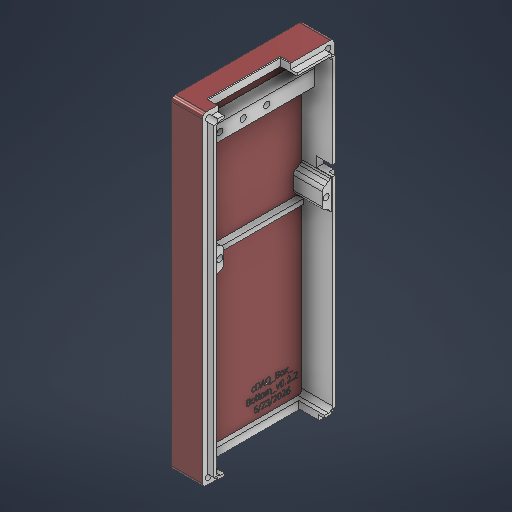
# Autodesk Inventor part: cDAQ_Box_Bottom_v0.2.2ipt
Saved by Autodesk Inventor 2027 (Build 310192000, 192)
## iProperties
Created: 2026-05-08
Part Number: cDAQ_Box_Bottom_v0.2.2ipt
Material: Generic
Document SubType Name: Modeling
Designer: giese
Density: 1 g/cm^3
Appearance: Default
Author: giese
Autodesk Inventor part; units mm, degrees
(part 1 of 2)
ref_plane "YZ Plane" through (0, 0, 0) normal (1, 0, 0) x (0, 1, 0)
ref_plane "XZ Plane" through (0, 0, 0) normal (0, 1, 0) x (-1, 0, 0)
ref_plane "XY Plane" through (0, 0, 0) normal (0, 0, 1) x (1, 0, 0)
sketch "Sketch1" plane through (0, 0, 0) normal (1, 0, 0) x (0, 1, 0)
  line L0 (37.5698, 55.7067) -> (-217.4462, 55.7067)
  line L1 (-217.4462, 55.7067) -> (-217.4462, -48.4333)
  line L2 (-217.4462, -48.4333) -> (37.5698, -48.4333)
  line L3 (37.5698, -48.4333) -> (37.5698, 55.7067)
  point P0 (0, 0)
  dimension "d0" = 104.14
  dimension "d1" = 255.016
  constraints: 8 end point, 2 parallel, 1 horizontal, 1 perpendicular
  measures "d0" distance of L2.end L0.start
  measures "d1" distance of L1.end L2.end
extrude "Extrusion1" add sketch "Sketch1" along normal blind 24.13
sketch "Sketch2" plane through (24.13, 0, 0) normal (1, 0, 0) x (0, 0, -1)
  line L0 (42.0833, 31.2198) -> (-49.3567, 31.2198)
  line L1 (-49.3567, 31.2198) -> (-49.3567, -211.0962)
  line L2 (-49.3567, -211.0962) -> (42.0833, -211.0962)
  line L3 (42.0833, -211.0962) -> (42.0833, 31.2198)
  line L4 (48.4333, 37.5698) -> (-55.7067, 37.5698) projected
  line L5 (-55.7067, 37.5698) -> (-55.7067, -217.4462) projected
  line L6 (-55.7067, -217.4462) -> (48.4333, -217.4462) projected
  line L7 (48.4333, -217.4462) -> (48.4333, 37.5698) projected
  point P0 (0, 0)
  dimension "d4" = 242.316
  dimension "d5" = 91.44
  dimension "d8" = 6.35
  dimension "d21" = 6.35
  dimension "d690" = 6.35
  dimension "d842" = 6.35
  constraints: 8 end point, 2 parallel, 1 horizontal, 1 perpendicular
  measures "d4" distance of L2.end L0.start
  measures "d5" distance of L0.start L0.end
  measures "d8" distance between parallel lines of L0 L4
  measures "d21" distance between parallel lines of L5 L1
  measures "d690" distance between parallel lines of L6 L2
  measures "d842" distance between parallel lines of L7 L3
extrude "Extrusion2" cut sketch "Sketch2" against normal blind 19.05 contours L3 L2 L1 L0
sketch "Sketch3" plane through (0, 0, 0) normal (-1, 0, 0) x (0, 0, 1)
  circle A0 centre (-4.1509, 9.6298) radius 2.4005
  circle A1 centre (14.3479, 9.6298) radius 2.4005
  circle A2 centre (32.8467, 9.6298) radius 2.4005
  line L0 (-48.4333, -217.4462) -> (-48.4333, 37.5698) projected
  line L1 (-48.4333, 37.5698) -> (55.7067, 37.5698) projected
  line L2 (55.7067, 37.5698) -> (55.7067, -217.4462) projected
  line L3 (49.3567, 31.2198) -> (-42.0833, 31.2198) projected
  point P0 (0, 0)
  point P1 (-0.896, -23.7433)
  point P2 (-45.1848, 27.0137)
  dimension "d9" = 18.4988
  dimension "d10" = 4.801
  dimension "d11" = 4.801
  dimension "d12" = 18.4988
  dimension "d13" = 36.9976
  dimension "d18" = 22.86
  dimension "d22" = 4.801
  dimension "d58" = 27.94
  constraints: 3 centre point
  measures "d9" distance of A0.centre A1.centre
  measures "d10" diameter of A1
  measures "d11" diameter of A2
  measures "d12" distance of A1.centre A2.centre
  measures "d13" distance of A0.centre A2.centre
  measures "d18" distance from line of L2 A2.centre
  measures "d22" diameter of A0
  measures "d58" distance from line of L1 A2.centre
extrude "Extrusion3" cut sketch "Sketch3" against normal blind 5.08
sketch "Sketch5" plane through (0, -217.4462, -48.4333) normal (0, 0, -1) x (-1, 0, 0)
  line L0 (-27.2034, 165.862) -> (-16.51, 165.862)
  line L1 (-16.51, 165.862) -> (-16.51, 173.862)
  line L2 (-16.51, 173.862) -> (-27.2034, 173.862)
  line L3 (-27.2034, 173.862) -> (-27.2034, 165.862)
  line L4 (0, 255.016) -> (-24.13, 255.016) projected
  line L5 (0, 0) -> (0, 255.016) projected
  line L6 (-24.13, 0) -> (-24.13, 255.016) projected
  line L7 (0, 0) -> (-24.13, 0) projected
  point P0 (0, 217.4462)
  point P1 (-21.8567, 173.862)
  point P2 (-21.8567, 165.862)
  dimension "d28" = 10.6934
  dimension "d30" = 8
  dimension "d31" = 16.51
  dimension "d215" = 3.0734
  dimension "d1133" = 165.862
  constraints: 8 end point, 2 midpoint, 2 parallel, 1 horizontal, 1 perpendicular
  measures "d28" distance between parallel lines of L1 L3
  measures "d30" distance of point (-21.857, 173.862) point (-21.857, 165.862)
  measures "d31" distance between parallel lines of L5 L1
  measures "d215" distance between parallel lines of L6 L3
  measures "d1133" distance between parallel lines of L7 L0
extrude "Extrusion4" cut sketch "Sketch5" against normal blind 24.13 contours L3 L2 L6 L0 | L6 L2 L1 L0
sketch "Sketch6" plane through (0, -217.4462, -48.4333) normal (0, -1, 0) x (1, 0, 0)
  line L0 (24.08, 55.136) -> (16.08, 55.136)
  line L1 (16.08, 45.136) -> (24.08, 45.136)
  line L2 (0, 104.14) -> (0, 0) projected
  line L3 (29.63, 53.1359) -> (29.63, 47.136)
  line L4 (24.08, 55.136) -> (29.63, 53.1359)
  line L5 (29.63, 47.136) -> (24.08, 45.136)
  line L6 (0, 0) -> (24.13, 0) projected
  line L7 (24.13, 97.79) -> (24.13, 6.35) projected
  line L8 (24.13, 41.9134) -> (24.13, 37.4697)
  line L9 (16.08, 55.136) -> (8.636, 55.136)
  line L10 (8.636, 55.136) -> (8.636, 45.136)
  line L11 (8.636, 45.136) -> (21.16, 45.136)
  point P0 (0, 48.4333)
  point P1 (20.08, 55.136)
  point P2 (20.08, 45.136)
  point P3 (16.08, 50.136)
  dimension "d39" = 6
  dimension "d48" = 55.136
  dimension "d221" = 0
  dimension "d223" = 2
  dimension "d224" = 2
  dimension "d225" = 5.5
  dimension "d227" = 5.55
  dimension "d672" = 8.636
  constraints: 18 end point, 2 horizontal, 2 midpoint, 2 parallel, 2 point on line, 1 perpendicular, 1 vertical
  measures "d39" distance of L3.start L3.end
  measures "d48" distance between parallel lines of L6 L0
  measures "d221" horizontal distance of L0.start L1.end
  measures "d223" vertical distance of L3.end L1.end
  measures "d224" vertical distance of L0.start L3.start
  measures "d225" distance between parallel lines of L3 L7
  measures "d227" distance from line of L1.end L3
  measures "d672" distance between parallel lines of L2 L10
extrude "Extrusion5" [suppressed]
sketch "Sketch7" plane through (0, 37.5698, 55.7067) normal (0, 1, 0) x (1, 0, 0)
  line L0 (31.0134, 69.85) -> (16.002, 69.85)
  line L1 (16.002, 69.85) -> (16.002, 12.7)
  line L2 (16.002, 12.7) -> (31.0134, 12.7)
  line L3 (31.0134, 12.7) -> (31.0134, 69.85)
  line L4 (0, 0) -> (24.13, 0) projected
  line L5 (0, 104.14) -> (0, 0) projected
  line L6 (24.13, 104.14) -> (24.13, 0) projected
  point P0 (0, 55.7067)
  point P1 (24.13, 69.85)
  point P2 (24.13, 12.7)
  dimension "d52" = 12.7
  dimension "d55" = 16.002
  dimension "d56" = 15.0114
  dimension "d57" = 6.8834
  dimension "d1195" = 69.85
  constraints: 8 end point, 2 parallel, 1 horizontal, 1 perpendicular
  measures "d52" distance between parallel lines of L4 L2
  measures "d55" distance between parallel lines of L5 L1
  measures "d56" distance between parallel lines of L3 L1
  measures "d57" distance between parallel lines of L6 L3
  measures "d1195" distance between parallel lines of L4 L0
extrude "Extrusion6" cut sketch "Sketch7" against normal blind 7.62
fillet "Fillet1" radius 3.175 4 edges at (12.065, 37.5698, -48.4333) (12.065, 37.5698, 55.7067) (12.065, -217.4462, -48.4333) (12.065, -217.4462, 55.7067)
sketch "Sketch8" plane through (0, 0, 0) normal (-1, 0, 0) x (0, 0, 1)
  line L0 (-5.9225, 6.0992) -> (-2.3919, 6.0992)
  line L1 (-5.9225, 13.1604) -> (-2.3919, 13.1604)
  line L2 (-5.9225, 6.0992) -> (-7.9609, 9.6298)
  line L3 (-5.9225, 13.1604) -> (-7.9609, 9.6298)
  line L4 (-2.3919, 6.0992) -> (-0.3536, 9.6298)
  line L5 (-2.3919, 13.1604) -> (-0.3536, 9.6298)
  circle A0 centre (-4.1509, 9.6298) radius 2.4005 projected
  line L6 (12.5763, 6.0992) -> (16.1069, 6.0992)
  line L7 (12.5763, 13.1604) -> (16.1069, 13.1604)
  line L8 (12.5763, 6.0992) -> (10.5379, 9.6298)
  line L9 (12.5763, 13.1604) -> (10.5379, 9.6298)
  line L10 (16.1069, 6.0992) -> (18.1453, 9.6298)
  line L11 (16.1069, 13.1604) -> (18.1453, 9.6298)
  circle A1 centre (14.3479, 9.6298) radius 2.4005 projected
  line L12 (31.0751, 6.0992) -> (29.0367, 9.6298)
  line L13 (31.0751, 13.1604) -> (29.0367, 9.6298)
  line L14 (31.0751, 6.0992) -> (34.6057, 6.0992)
  line L15 (31.0751, 13.1604) -> (34.6057, 13.1604)
  line L16 (34.6057, 6.0992) -> (36.6441, 9.6298)
  line L17 (34.6057, 13.1604) -> (36.6441, 9.6298)
  circle A2 centre (32.8467, 9.6298) radius 2.4005 projected
  point P0 (-4.1572, 6.0992)
  point P1 (14.3416, 6.0992)
  point P2 (32.8404, 6.0992)
  point P3 (-7.9609, 9.6298)
  point P4 (-0.3536, 9.6298)
  point P5 (18.1453, 9.6298)
  point P6 (10.5379, 9.6298)
  point P7 (36.6441, 9.6298)
  point P8 (29.0367, 9.6298)
  dimension "d60" = 7.0612
  dimension "d61" = 120
  dimension "d62" = 120
  dimension "d63" = 120
  dimension "d64" = 120
  dimension "d65" = 3.5306
  dimension "d66" = 3.5306
  dimension "d67" = 3.5306
  dimension "d68" = 3.5306
  dimension "d69" = 3.5306
  dimension "d70" = 3.5306
  dimension "d71" = 0
  dimension "d72" = 7.6074
  dimension "d73" = 3.81
  dimension "d74" = 0
  dimension "d75" = 7.0612
  dimension "d76" = 120
  dimension "d77" = 120
  dimension "d78" = 120
  dimension "d79" = 120
  dimension "d80" = 3.5306
  dimension "d81" = 3.5306
  dimension "d82" = 3.5306
  dimension "d83" = 3.5306
  dimension "d84" = 3.5306
  dimension "d85" = 3.5306
  dimension "d86" = 0
  dimension "d87" = 7.6074
  dimension "d91" = 0
  dimension "d92" = 3.81
  dimension "d93" = 7.0612
  dimension "d94" = 120
  dimension "d95" = 120
  dimension "d96" = 120
  dimension "d97" = 120
  dimension "d98" = 3.5306
  dimension "d99" = 3.5306
  dimension "d100" = 3.5306
  dimension "d101" = 3.5306
  dimension "d102" = 3.5306
  dimension "d103" = 3.5306
  dimension "d104" = 0
  dimension "d105" = 7.6074
  dimension "d108" = 0
  dimension "d109" = 3.81
  constraints: 36 end point, 6 horizontal, 3 midpoint
  measures "d60" distance from line of point (-4.157, 6.099) L1
  measures "d61" angle of L0 L2
  measures "d62" angle of L1 L3
  measures "d63" angle of L4 L0
  measures "d64" angle of L5 L1
  measures "d65" distance of L0.start L0.end
  measures "d66" distance of L1.start L1.end
  measures "d67" vertical distance of L1.start L3.end
  measures "d68" vertical distance of L0.start L2.end
  measures "d69" vertical distance of L1.end L5.end
  measures "d70" vertical distance of L0.end L4.end
  measures "d71" horizontal distance of L0.start L1.start
  measures "d72" distance of L4.end L2.end
  measures "d73" distance of A0.centre L2.end
  measures "d74" vertical distance of A0.centre L4.end
  measures "d75" distance from line of point (14.342, 6.099) L7
  measures "d76" angle of L6 L8
  measures "d77" angle of L7 L9
  measures "d78" angle of L10 L6
  measures "d79" angle of L11 L7
  measures "d80" distance of L8.start L6.end
  measures "d81" distance of L9.start L7.end
  measures "d82" vertical distance of L9.start L9.end
  measures "d83" vertical distance of L8.start L8.end
  measures "d84" vertical distance of L7.end L11.end
  measures "d85" vertical distance of L6.end L10.end
  measures "d86" horizontal distance of L8.start L9.start
  measures "d87" distance of L10.end L8.end
  measures "d91" vertical distance of A1.centre L8.end
  measures "d92" distance of A1.centre L8.end
  measures "d93" distance from line of point (32.84, 6.099) L15
  measures "d94" angle of L14 L12
  measures "d95" angle of L15 L13
  measures "d96" angle of L16 L14
  measures "d97" angle of L17 L15
  measures "d98" distance of L12.start L16.start
  measures "d99" distance of L15.start L15.end
  measures "d100" vertical distance of L15.start L13.end
  measures "d101" vertical distance of L12.start L12.end
  measures "d102" vertical distance of L15.end L17.end
  measures "d103" vertical distance of L16.start L16.end
  measures "d104" horizontal distance of L12.start L15.start
  measures "d105" distance of L16.end L12.end
  measures "d108" vertical distance of A2.centre L12.end
  measures "d109" distance of A2.centre L12.end
extrude "Extrusion7" cut sketch "Sketch8" against normal blind 4 contours L2 L3 L1 L5 L4 L0 | A0 | L8 L9 L7 L11 L10 L6 | A1 | L12 L13 L15 L17 L16 L14 | A2
sketch "Sketch9" plane through (5.08, 0, 0) normal (1, 0, 0) x (0, 0, -1)
  arc A0 (24.8089, -180.8044) -> (19.3527, -180.8044) centre (22.0808, -178.3302) ccw
  line L0 (45.2583, 37.5698) -> (14.1433, 37.5698) projected
  line L1 (42.0833, 31.2198) -> (42.0833, -43.5842) projected
  arc A1 (20.1758, -185.9502) -> (23.9858, -185.9502) centre (22.0808, -185.9502) ccw
  line L2 (23.9858, -185.9502) -> (23.9858, -182.9374)
  line L3 (20.1758, -185.9502) -> (20.1758, -182.9374)
  arc A2 (24.8089, -180.8044) -> (23.9858, -182.9374) centre (27.1608, -182.9374) ccw
  arc A3 (20.1758, -182.9374) -> (19.3527, -180.8044) centre (17.0008, -182.9374) ccw
  arc A4 (-25.9911, -180.8044) -> (-31.4473, -180.8045) centre (-28.7192, -178.3302) ccw
  arc A5 (-30.6242, -185.9366) -> (-26.8142, -185.9502) centre (-28.7192, -185.9502) ccw
  line L4 (-26.8142, -185.9502) -> (-26.8142, -182.9374)
  line L5 (-30.6242, -185.9366) -> (-30.6242, -182.9374)
  arc A6 (-25.9911, -180.8044) -> (-26.8142, -182.9374) centre (-23.6392, -182.9374) ccw
  arc A7 (-30.6242, -182.9374) -> (-31.4473, -180.8045) centre (-33.7992, -182.9374) ccw
  line L6 (-43.0067, 37.5698) -> (-52.5317, 37.5698) projected
  line L7 (-49.3567, -211.0962) -> (-49.3567, 31.2198) projected
  point P0 (0, 0)
  point P1 (42.0833, -211.0962)
  point P2 (23.9858, -181.4823)
  point P3 (20.1758, -181.4823)
  point P4 (-26.8142, -181.4823)
  point P5 (-30.6242, -181.4823)
  point P6 (-49.3567, 31.2198)
  point P7 (-46.8167, -217.4462)
  dimension "d112" = 215.9
  dimension "d114" = 7.366
  dimension "d116" = 3.81
  dimension "d117" = 223.52
  dimension "d118" = 3.175
  dimension "d119" = 7.366
  dimension "d120" = 3.81
  dimension "d121" = 3.175
  dimension "d122" = 215.9
  dimension "d123" = 223.52
  dimension "d125" = 0
  dimension "d128" = 50.8
  dimension "d129" = 20.0025
  dimension "d130" = 0
  constraints: 20 point on circle, 8 centre point, 8 end point, 8 tangent, 4 point on line, 2 equal radius, 2 parallel, 2 vertical, 1 other
  measures "d112" distance from line of L0 A0.centre
  measures "d114" diameter of A0
  measures "d116" diameter of A1
  measures "d117" distance from line of L0 A1.centre
  measures "d118" radius of A2
  measures "d119" diameter of A4
  measures "d120" diameter of A5
  measures "d121" radius of A6
  measures "d122" distance from line of A4.centre L6
  measures "d123" distance from line of L6 A5.centre
  measures "d125" horizontal distance of A5.centre A4.centre
  measures "d128" distance of A5.centre A1.centre
  measures "d129" distance from line of L1 A0.centre
  measures "d130" horizontal distance of A0.centre A1.centre
extrude "Extrusion8" [suppressed]
sketch "Sketch10" plane through (24.13, 0, 0) normal (1, 0, 0) x (0, 0, -1)
  line L0 (-49.3567, 31.2198) -> (42.0833, 31.2198) projected
  line L1 (-49.3567, 31.2198) -> (42.0833, 31.2198)
  line L2 (42.0833, 33.2264) -> (-46.8167, 33.2264)
  line L3 (-46.8167, 33.2264) -> (-51.3633, 33.2264)
  line L4 (-51.3633, 33.2264) -> (-51.3633, -213.1028)
  line L5 (-51.3633, -213.1028) -> (44.0899, -213.1028)
  line L6 (44.0899, -213.1028) -> (44.0899, 33.2264)
  line L7 (44.0899, 33.2264) -> (41.9392, 33.2264)
  line L8 (42.0833, 31.2198) -> (42.0833, -43.5842) projected
  line L9 (-49.3567, -211.0962) -> (-49.3567, 31.2198) projected
  line L10 (42.0833, -211.0962) -> (-49.3567, -211.0962) projected
  line L11 (45.2583, 37.5698) -> (14.1433, 37.5698) projected
  line L12 (42.0833, 31.2198) -> (42.0833, -211.0962)
  line L13 (42.0833, -211.0962) -> (-49.3567, -211.0962)
  line L14 (-52.5317, -217.4462) -> (45.2583, -217.4462) projected
  line L15 (-49.3567, -211.0962) -> (-49.3567, 31.2198)
  line L16 (-49.3567, 31.2198) -> (42.0833, 31.2198)
  point P0 (-46.8167, -217.4462)
  dimension "d202" = 2.0066
  dimension "d203" = 2.0066
  dimension "d204" = 2.0066
  dimension "d205" = 2.0066
  dimension "d208" = 4.3434
  constraints: 22 end point, 5 perpendicular, 3 point on line, 2 parallel, 1 collinear, 1 horizontal, 1 other
  measures "d202" distance between parallel lines of L0 L2
  measures "d203" distance between parallel lines of L6 L8
  measures "d205" distance between parallel lines of L5 L10
  measures "d208" distance between parallel lines of L11 L2
extrude "Extrusion9" add sketch "Sketch10" along normal blind 5
fillet "Fillet2" radius 3.175 8 edges at (17.105, 31.2198, -42.0833) (17.105, 31.2198, 49.3567) (17.105, -211.0962, 49.3567) (17.105, -211.0962, -42.0833) (26.63, 33.2264, -44.0899) (26.63, 33.2264, 51.3633) (26.63, -213.1028, -44.0899) (26.63, -213.1028, 51.3633)
sketch "Sketch13" plane through (29.13, 0, 0) normal (1, 0, 0) x (0, 0, -1)
  arc A0 (44.0833, 30.0448) -> (40.9083, 33.2198) centre (40.9083, 30.0448) ccw projected
  arc A1 (-45.6417, 33.2198) -> (-48.8167, 30.0448) centre (-45.6417, 30.0448) ccw projected
  arc A2 (40.9083, -212.0802) -> (44.0833, -208.9052) centre (40.9083, -208.9052) ccw projected
  arc A3 (-48.8167, -208.9052) -> (-45.6417, -212.0802) centre (-45.6417, -208.9052) ccw projected
  line L0 (-43.0067, 37.5698) -> (-52.5317, 37.5698) projected
  line L1 (-55.7067, 34.3948) -> (-55.7067, -214.2712) projected
  line L2 (-52.5317, -217.4462) -> (45.2583, -217.4462) projected
  arc A4 (-48.8167, -208.9052) -> (-45.6417, -212.0802) centre (-45.6417, -208.9052) ccw projected
  circle A5 centre (-50.6267, -212.3662) radius 2.4005
  circle A6 centre (43.3533, -212.3662) radius 2.4005
  line L3 (48.4333, -214.2712) -> (48.4333, 34.3948) projected
  circle A7 centre (43.3533, 32.4898) radius 2.4005
  line L4 (45.2583, 37.5698) -> (14.1433, 37.5698) projected
  circle A8 centre (-50.6267, 32.4898) radius 2.4005
  arc A9 (41.4904, -28.6131) -> (38.3154, -25.4381) centre (38.3154, -28.6131) ccw
  circle A10 centre (38.2733, -64.0302) radius 2.4005
  circle A11 centre (-45.5467, -64.0302) radius 2.4005
  point P0 (0, 0)
  point P1 (-47.8868, 32.2898)
  point P2 (-47.8868, -211.1503)
  point P3 (-47.8868, -211.1503)
  point P4 (45.8404, -24.2631)
  point P5 (42.6654, -21.0881)
  dimension "d178" = 5.08
  dimension "d179" = 5.08
  dimension "d180" = 4.801
  dimension "d181" = 5.08
  dimension "d182" = 5.08
  dimension "d183" = 4.801
  dimension "d184" = 4.801
  dimension "d185" = 5.08
  dimension "d186" = 5.08
  dimension "d187" = 4.801
  dimension "d188" = 5.08
  dimension "d189" = 5.08
  dimension "d326" = 4.801
  dimension "d327" = 10.16
  dimension "d328" = 101.6
  dimension "d329" = 4.801
  dimension "d330" = 10.16
  dimension "d331" = 101.6
  constraints: 7 centre point, 5 point on circle
  measures "d178" distance from line of L1 A5.centre
  measures "d179" distance from line of L2 A5.centre
  measures "d180" diameter of A5
  measures "d181" distance from line of L2 A6.centre
  measures "d182" distance from line of L3 A6.centre
  measures "d183" diameter of A6
  measures "d184" diameter of A7
  measures "d185" distance from line of L3 A7.centre
  measures "d186" distance from line of L4 A7.centre
  measures "d187" diameter of A8
  measures "d188" distance from line of L0 A8.centre
  measures "d189" distance from line of L1 A8.centre
  measures "d326" diameter of A10
  measures "d327" distance from line of L3 A10.centre
  measures "d328" distance from line of A10.centre L4
  measures "d329" diameter of A11
  measures "d330" distance from line of L1 A11.centre
  measures "d331" distance from line of L0 A11.centre
extrude "Extrusion11" cut sketch "Sketch13" against normal blind 25.4
sketch "Sketch14" plane through (5.08, 0, 0) normal (1, 0, 0) x (0, 0, -1)
  line L0 (8.8875, -186.6885) -> (28.1042, -186.6885) construction
  line L1 (28.1042, -186.6885) -> (28.1042, -184.7391) construction
  line L2 (28.1042, -184.7391) -> (8.8875, -184.7391) construction
  line L3 (8.8875, -184.7391) -> (8.8875, -186.6885) construction
  spline S0 degree 2 poles (3.9907, -191.4347) (3.635, -191.4347) (3.0459, -191.2161) (2.8347, -190.9938) knots 0 0 0 1 2 2 2
  spline S1 degree 2 poles (2.8347, -190.9938) (2.6236, -190.7752) (2.3901, -190.1008) (2.3901, -189.6488) knots 0 0 0 1 2 2 2
  spline S2 degree 2 poles (2.3901, -189.6488) (2.3901, -189.1968) (2.631, -188.5373) (2.8347, -188.315) knots 0 0 0 1 2 2 2
  spline S3 degree 2 poles (2.8347, -188.315) (3.0385, -188.089) (3.6424, -187.8482) (3.9907, -187.8482) knots 0 0 0 1 2 2 2
  spline S4 degree 2 poles (3.9907, -187.8482) (4.2723, -187.8482) (4.7984, -188.0075) (5.0022, -188.1112) knots 0 0 0 1 2 2 2
  line L4 (5.0022, -188.1112) -> (5.0022, -188.7596)
  line L5 (5.0022, -188.7596) -> (4.9688, -188.7596)
  spline S5 degree 2 poles (4.9688, -188.7596) (4.9058, -188.7078) (4.7132, -188.5744) (4.5761, -188.504) knots 0 0 0 1 2 2 2
  spline S6 degree 2 poles (4.5761, -188.504) (4.4538, -188.4447) (4.1278, -188.3521) (3.9796, -188.3521) knots 0 0 0 1 2 2 2
  spline S7 degree 2 poles (3.9796, -188.3521) (3.5313, -188.3521) (2.9866, -189.0301) (2.9866, -189.6488) knots 0 0 0 1 2 2 2
  spline S8 degree 2 poles (2.9866, -189.6488) (2.9866, -190.2528) (3.5128, -190.9308) (3.9796, -190.9308) knots 0 0 0 1 2 2 2
  spline S9 degree 2 poles (3.9796, -190.9308) (4.2612, -190.9308) (4.7725, -190.6974) (4.9688, -190.5158) knots 0 0 0 1 2 2 2
  line L6 (4.9688, -190.5158) -> (5.0022, -190.5158)
  line L7 (5.0022, -190.5158) -> (5.0022, -191.1642)
  spline S10 degree 2 poles (5.0022, -191.1642) (4.917, -191.2049) (4.6576, -191.3198) (4.5539, -191.3457) knots 0 0 0 1 2 2 2
  spline S11 degree 2 poles (4.5539, -191.3457) (4.4057, -191.3902) (4.1723, -191.4347) (3.9907, -191.4347) knots 0 0 0 1 2 2 2
  spline S12 degree 2 poles (9.1777, -189.0746) (9.1777, -189.7007) (8.6702, -190.7085) (8.2441, -190.9901) knots 0 0 0 1 2 2 2
  spline S13 degree 2 poles (8.2441, -190.9901) (7.8958, -191.2087) (7.1807, -191.3569) (6.625, -191.3569) knots 0 0 0 1 2 2 2
  line L8 (6.625, -191.3569) -> (5.5728, -191.3569)
  line L9 (5.5728, -191.3569) -> (5.5728, -186.7849)
  line L10 (5.5728, -186.7849) -> (6.6139, -186.7849)
  spline S14 degree 2 poles (6.6139, -186.7849) (7.2585, -186.7849) (7.9921, -186.9775) (8.2515, -187.1479) knots 0 0 0 1 2 2 2
  spline S15 degree 2 poles (8.2515, -187.1479) (8.6924, -187.4406) (9.1777, -188.4077) (9.1777, -189.0746) knots 0 0 0 1 2 2 2
  spline S16 degree 2 poles (8.5442, -189.0671) (8.5442, -188.541) (8.1959, -187.7963) (7.8513, -187.5851) knots 0 0 0 1 2 2 2
  spline S17 degree 2 poles (7.8513, -187.5851) (7.6068, -187.4406) (7.0548, -187.311) (6.6435, -187.311) knots 0 0 0 1 2 2 2
  line L11 (6.6435, -187.311) -> (6.1804, -187.311)
  line L12 (6.1804, -187.311) -> (6.1804, -190.8307)
  line L13 (6.1804, -190.8307) -> (6.6435, -190.8307)
  spline S18 degree 2 poles (6.6435, -190.8307) (7.0474, -190.8307) (7.6587, -190.7011) (7.9069, -190.5269) knots 0 0 0 1 2 2 2
  spline S19 degree 2 poles (7.9069, -190.5269) (8.2255, -190.312) (8.5442, -189.6007) (8.5442, -189.0671) knots 0 0 0 1 2 2 2
  line L14 (9.3445, -191.3569) -> (10.8858, -186.7849)
  line L15 (10.8858, -186.7849) -> (11.6342, -186.7849)
  line L16 (11.6342, -186.7849) -> (13.1755, -191.3569)
  line L17 (13.1755, -191.3569) -> (12.5345, -191.3569)
  line L18 (12.5345, -191.3569) -> (12.1195, -190.0786)
  line L19 (12.1195, -190.0786) -> (10.3745, -190.0786)
  line L20 (10.3745, -190.0786) -> (9.9595, -191.3569)
  line L21 (9.9595, -191.3569) -> (9.3445, -191.3569)
  line L22 (11.9528, -189.5599) -> (11.2451, -187.4073)
  line L23 (11.2451, -187.4073) -> (10.5412, -189.5599)
  line L24 (10.5412, -189.5599) -> (11.9528, -189.5599)
  spline S20 degree 2 poles (17.4066, -192.4758) (17.2399, -192.5165) (16.8768, -192.561) (16.6952, -192.561) knots 0 0 0 1 2 2 2
  spline S21 degree 2 poles (16.6952, -192.561) (16.1802, -192.561) (15.5393, -191.9867) (15.5096, -191.4532) knots 0 0 0 1 2 2 2
  spline S22 degree 2 poles (15.5096, -191.4532) (15.4689, -191.4532) (15.3985, -191.4532) (15.3688, -191.4532) knots 0 0 0 1 2 2 2
  spline S23 degree 2 poles (15.3688, -191.4532) (14.9057, -191.4532) (14.161, -191.1383) (13.8942, -190.8307) knots 0 0 0 1 2 2 2
  spline S24 degree 2 poles (13.8942, -190.8307) (13.6312, -190.5269) (13.3496, -189.6377) (13.3496, -189.0746) knots 0 0 0 1 2 2 2
  spline S25 degree 2 poles (13.3496, -189.0746) (13.3496, -188.4966) (13.6349, -187.6222) (13.8979, -187.311) knots 0 0 0 1 2 2 2
  spline S26 degree 2 poles (13.8979, -187.311) (14.1647, -187.0034) (14.9094, -186.6885) (15.3688, -186.6885) knots 0 0 0 1 2 2 2
  spline S27 degree 2 poles (15.3688, -186.6885) (15.8357, -186.6885) (16.5841, -187.0146) (16.8434, -187.311) knots 0 0 0 1 2 2 2
  spline S28 degree 2 poles (16.8434, -187.311) (17.1028, -187.6111) (17.3918, -188.504) (17.3918, -189.0746) knots 0 0 0 1 2 2 2
  spline S29 degree 2 poles (17.3918, -189.0746) (17.3918, -189.9638) (16.6989, -191.1197) (16.095, -191.3235) knots 0 0 0 1 2 2 2
  spline S30 degree 2 poles (16.095, -191.3235) (16.1098, -191.4939) (16.1988, -191.7681) (16.2692, -191.8459) knots 0 0 0 1 2 2 2
  spline S31 degree 2 poles (16.2692, -191.8459) (16.3544, -191.9422) (16.5878, -192.0312) (16.7953, -192.0312) knots 0 0 0 1 2 2 2
  spline S32 degree 2 poles (16.7953, -192.0312) (16.9175, -192.0312) (17.251, -191.9534) (17.3251, -191.9237) knots 0 0 0 1 2 2 2
  line L25 (17.3251, -191.9237) -> (17.4066, -191.9237)
  line L26 (17.4066, -191.9237) -> (17.4066, -192.4758)
  spline S33 degree 2 poles (16.7582, -189.0746) (16.7582, -188.6188) (16.5619, -187.9186) (16.384, -187.6889) knots 0 0 0 1 2 2 2
  spline S34 degree 2 poles (16.384, -187.6889) (16.2025, -187.4518) (15.6912, -187.2146) (15.3725, -187.2146) knots 0 0 0 1 2 2 2
  spline S35 degree 2 poles (15.3725, -187.2146) (15.0428, -187.2146) (14.5463, -187.4443) (14.3574, -187.6889) knots 0 0 0 1 2 2 2
  spline S36 degree 2 poles (14.3574, -187.6889) (14.1758, -187.9223) (13.9832, -188.63) (13.9832, -189.0746) knots 0 0 0 1 2 2 2
  spline S37 degree 2 poles (13.9832, -189.0746) (13.9832, -189.9749) (14.739, -190.9345) (15.3725, -190.9345) knots 0 0 0 1 2 2 2
  spline S38 degree 2 poles (15.3725, -190.9345) (16.0061, -190.9345) (16.7582, -189.9749) (16.7582, -189.0746) knots 0 0 0 1 2 2 2
  line L27 (21.0746, -192.2757) -> (17.5474, -192.2757)
  line L28 (17.5474, -192.2757) -> (17.5474, -191.8793)
  line L29 (17.5474, -191.8793) -> (21.0746, -191.8793)
  line L30 (21.0746, -191.8793) -> (21.0746, -192.2757)
  spline S39 degree 2 poles (24.5906, -189.9526) (24.5906, -190.2935) (24.3313, -190.8159) (24.1164, -190.9863) knots 0 0 0 1 2 2 2
  spline S40 degree 2 poles (24.1164, -190.9863) (23.857, -191.1864) (23.2679, -191.3569) (22.8011, -191.3569) knots 0 0 0 1 2 2 2
  line L31 (22.8011, -191.3569) -> (21.4895, -191.3569)
  line L32 (21.4895, -191.3569) -> (21.4895, -186.7849)
  line L33 (21.4895, -186.7849) -> (22.7011, -186.7849)
  spline S41 degree 2 poles (22.7011, -186.7849) (23.1901, -186.7849) (23.6792, -186.8478) (23.9015, -186.9701) knots 0 0 0 1 2 2 2
  spline S42 degree 2 poles (23.9015, -186.9701) (24.1497, -187.0998) (24.3757, -187.5259) (24.3757, -187.8148) knots 0 0 0 1 2 2 2
  spline S43 degree 2 poles (24.3757, -187.8148) (24.3757, -188.1372) (24.0349, -188.6485) (23.7348, -188.793) knots 0 0 0 1 2 2 2
  line L34 (23.7348, -188.793) -> (23.7348, -188.8152)
  spline S44 degree 2 poles (23.7348, -188.8152) (24.1423, -188.9264) (24.5906, -189.5155) (24.5906, -189.9526) knots 0 0 0 1 2 2 2
  spline S45 degree 2 poles (23.9571, -189.9786) (23.9571, -189.7192) (23.8089, -189.3858) (23.5866, -189.2672) knots 0 0 0 1 2 2 2
  spline S46 degree 2 poles (23.5866, -189.2672) (23.4421, -189.1931) (23.1012, -189.1487) (22.7863, -189.1487) knots 0 0 0 1 2 2 2
  line L35 (22.7863, -189.1487) -> (22.0972, -189.1487)
  line L36 (22.0972, -189.1487) -> (22.0972, -190.8381)
  line L37 (22.0972, -190.8381) -> (22.5899, -190.8381)
  spline S47 degree 2 poles (22.5899, -190.8381) (22.9901, -190.8381) (23.4495, -190.764) (23.6273, -190.6455) knots 0 0 0 1 2 2 2
  spline S48 degree 2 poles (23.6273, -190.6455) (23.7978, -190.5232) (23.9571, -190.2194) (23.9571, -189.9786) knots 0 0 0 1 2 2 2
  spline S49 degree 2 poles (23.7422, -187.9001) (23.7422, -187.737) (23.631, -187.4925) (23.5088, -187.4221) knots 0 0 0 1 2 2 2
  spline S50 degree 2 poles (23.5088, -187.4221) (23.3606, -187.3406) (23.0012, -187.3036) (22.6788, -187.3036) knots 0 0 0 1 2 2 2
  line L38 (22.6788, -187.3036) -> (22.0972, -187.3036)
  line L39 (22.0972, -187.3036) -> (22.0972, -188.6411)
  line L40 (22.0972, -188.6411) -> (22.7863, -188.6411)
  spline S51 degree 2 poles (22.7863, -188.6411) (23.0716, -188.6411) (23.342, -188.5818) (23.4865, -188.4892) knots 0 0 0 1 2 2 2
  spline S52 degree 2 poles (23.4865, -188.4892) (23.6273, -188.4002) (23.7422, -188.115) (23.7422, -187.9001) knots 0 0 0 1 2 2 2
  spline S53 degree 2 poles (27.9696, -189.6414) (27.9696, -190.5084) (27.136, -191.4532) (26.4394, -191.4532) knots 0 0 0 1 2 2 2
  spline S54 degree 2 poles (26.4394, -191.4532) (25.7244, -191.4532) (24.9056, -190.4788) (24.9056, -189.6414) knots 0 0 0 1 2 2 2
  spline S55 degree 2 poles (24.9056, -189.6414) (24.9056, -188.7819) (25.7503, -187.8297) (26.4394, -187.8297) knots 0 0 0 1 2 2 2
  spline S56 degree 2 poles (26.4394, -187.8297) (27.136, -187.8297) (27.9696, -188.7782) (27.9696, -189.6414) knots 0 0 0 1 2 2 2
  spline S57 degree 2 poles (27.3731, -189.6414) (27.3731, -188.9745) (26.8878, -188.3261) (26.4394, -188.3261) knots 0 0 0 1 2 2 2
  spline S58 degree 2 poles (26.4394, -188.3261) (25.9911, -188.3261) (25.5021, -188.9745) (25.5021, -189.6414) knots 0 0 0 1 2 2 2
  spline S59 degree 2 poles (25.5021, -189.6414) (25.5021, -190.2898) (25.9911, -190.9567) (26.4394, -190.9567) knots 0 0 0 1 2 2 2
  spline S60 degree 2 poles (26.4394, -190.9567) (26.8841, -190.9567) (27.3731, -190.3009) (27.3731, -189.6414) knots 0 0 0 1 2 2 2
  line L41 (31.2263, -191.3569) -> (30.5187, -191.3569)
  line L42 (30.5187, -191.3569) -> (29.685, -190.0675)
  line L43 (29.685, -190.0675) -> (28.8292, -191.3569)
  line L44 (28.8292, -191.3569) -> (28.1734, -191.3569)
  line L45 (28.1734, -191.3569) -> (29.3627, -189.6562)
  line L46 (29.3627, -189.6562) -> (28.1845, -187.926)
  line L47 (28.1845, -187.926) -> (28.8922, -187.926)
  line L48 (28.8922, -187.926) -> (29.7221, -189.2042)
  line L49 (29.7221, -189.2042) -> (30.5705, -187.926)
  line L50 (30.5705, -187.926) -> (31.2263, -187.926)
  line L51 (31.2263, -187.926) -> (30.0444, -189.6192)
  line L52 (30.0444, -189.6192) -> (31.2263, -191.3569)
  line L53 (34.735, -192.2757) -> (31.2078, -192.2757)
  line L54 (31.2078, -192.2757) -> (31.2078, -191.8793)
  line L55 (31.2078, -191.8793) -> (34.735, -191.8793)
  line L56 (34.735, -191.8793) -> (34.735, -192.2757)
  spline S61 degree 2 poles (1.7195, -197.4803) (1.7195, -197.8212) (1.4602, -198.3436) (1.2453, -198.514) knots 0 0 0 1 2 2 2
  spline S62 degree 2 poles (1.2453, -198.514) (0.9859, -198.7141) (0.3968, -198.8845) (-0.07, -198.8845) knots 0 0 0 1 2 2 2
  line L57 (-0.07, -198.8845) -> (-1.3816, -198.8845)
  line L58 (-1.3816, -198.8845) -> (-1.3816, -194.3125)
  line L59 (-1.3816, -194.3125) -> (-0.17, -194.3125)
  spline S63 degree 2 poles (-0.17, -194.3125) (0.319, -194.3125) (0.8081, -194.3755) (1.0304, -194.4978) knots 0 0 0 1 2 2 2
  spline S64 degree 2 poles (1.0304, -194.4978) (1.2786, -194.6275) (1.5046, -195.0535) (1.5046, -195.3425) knots 0 0 0 1 2 2 2
  spline S65 degree 2 poles (1.5046, -195.3425) (1.5046, -195.6649) (1.1638, -196.1762) (0.8637, -196.3207) knots 0 0 0 1 2 2 2
  line L60 (0.8637, -196.3207) -> (0.8637, -196.3429)
  spline S66 degree 2 poles (0.8637, -196.3429) (1.2712, -196.454) (1.7195, -197.0431) (1.7195, -197.4803) knots 0 0 0 1 2 2 2
  spline S67 degree 2 poles (1.086, -197.5063) (1.086, -197.2469) (0.9378, -196.9135) (0.7155, -196.7949) knots 0 0 0 1 2 2 2
  spline S68 degree 2 poles (0.7155, -196.7949) (0.571, -196.7208) (0.2301, -196.6763) (-0.0848, -196.6763) knots 0 0 0 1 2 2 2
  line L61 (-0.0848, -196.6763) -> (-0.774, -196.6763)
  line L62 (-0.774, -196.6763) -> (-0.774, -198.3658)
  line L63 (-0.774, -198.3658) -> (-0.2812, -198.3658)
  spline S69 degree 2 poles (-0.2812, -198.3658) (0.119, -198.3658) (0.5784, -198.2917) (0.7562, -198.1732) knots 0 0 0 1 2 2 2
  spline S70 degree 2 poles (0.7562, -198.1732) (0.9267, -198.0509) (1.086, -197.7471) (1.086, -197.5063) knots 0 0 0 1 2 2 2
  spline S71 degree 2 poles (0.8711, -195.4277) (0.8711, -195.2647) (0.7599, -195.0202) (0.6377, -194.9498) knots 0 0 0 1 2 2 2
  spline S72 degree 2 poles (0.6377, -194.9498) (0.4895, -194.8683) (0.1301, -194.8312) (-0.1923, -194.8312) knots 0 0 0 1 2 2 2
  line L64 (-0.1923, -194.8312) -> (-0.774, -194.8312)
  line L65 (-0.774, -194.8312) -> (-0.774, -196.1687)
  line L66 (-0.774, -196.1687) -> (-0.0848, -196.1687)
  spline S73 degree 2 poles (-0.0848, -196.1687) (0.2005, -196.1687) (0.4709, -196.1095) (0.6154, -196.0168) knots 0 0 0 1 2 2 2
  spline S74 degree 2 poles (0.6154, -196.0168) (0.7562, -195.9279) (0.8711, -195.6426) (0.8711, -195.4277) knots 0 0 0 1 2 2 2
  spline S75 degree 2 poles (5.0985, -197.1691) (5.0985, -198.0361) (4.2649, -198.9809) (3.5683, -198.9809) knots 0 0 0 1 2 2 2
  spline S76 degree 2 poles (3.5683, -198.9809) (2.8533, -198.9809) (2.0345, -198.0064) (2.0345, -197.1691) knots 0 0 0 1 2 2 2
  spline S77 degree 2 poles (2.0345, -197.1691) (2.0345, -196.3095) (2.8792, -195.3573) (3.5683, -195.3573) knots 0 0 0 1 2 2 2
  spline S78 degree 2 poles (3.5683, -195.3573) (4.2649, -195.3573) (5.0985, -196.3058) (5.0985, -197.1691) knots 0 0 0 1 2 2 2
  spline S79 degree 2 poles (4.502, -197.1691) (4.502, -196.5022) (4.0166, -195.8538) (3.5683, -195.8538) knots 0 0 0 1 2 2 2
  spline S80 degree 2 poles (3.5683, -195.8538) (3.12, -195.8538) (2.631, -196.5022) (2.631, -197.1691) knots 0 0 0 1 2 2 2
  spline S81 degree 2 poles (2.631, -197.1691) (2.631, -197.8175) (3.12, -198.4844) (3.5683, -198.4844) knots 0 0 0 1 2 2 2
  spline S82 degree 2 poles (3.5683, -198.4844) (4.0129, -198.4844) (4.502, -197.8286) (4.502, -197.1691) knots 0 0 0 1 2 2 2
  spline S83 degree 2 poles (6.7287, -198.9512) (6.2582, -198.9512) (5.7284, -198.414) (5.7284, -197.8323) knots 0 0 0 1 2 2 2
  line L67 (5.7284, -197.8323) -> (5.7284, -195.9316)
  line L68 (5.7284, -195.9316) -> (5.3393, -195.9316)
  line L69 (5.3393, -195.9316) -> (5.3393, -195.4537)
  line L70 (5.3393, -195.4537) -> (5.7284, -195.4537)
  line L71 (5.7284, -195.4537) -> (5.7284, -194.4681)
  line L72 (5.7284, -194.4681) -> (6.3063, -194.4681)
  line L73 (6.3063, -194.4681) -> (6.3063, -195.4537)
  line L74 (6.3063, -195.4537) -> (7.3697, -195.4537)
  line L75 (7.3697, -195.4537) -> (7.3697, -195.9316)
  line L76 (7.3697, -195.9316) -> (6.3063, -195.9316)
  line L77 (6.3063, -195.9316) -> (6.3063, -197.5655)
  spline S84 degree 2 poles (6.3063, -197.5655) (6.3063, -197.8249) (6.3249, -198.1102) (6.3879, -198.2324) knots 0 0 0 1 2 2 2
  spline S85 degree 2 poles (6.3879, -198.2324) (6.4397, -198.3399) (6.6731, -198.4473) (6.8732, -198.4473) knots 0 0 0 1 2 2 2
  spline S86 degree 2 poles (6.8732, -198.4473) (7.014, -198.4473) (7.2771, -198.3621) (7.3363, -198.3362) knots 0 0 0 1 2 2 2
  line L78 (7.3363, -198.3362) -> (7.3697, -198.3362)
  line L79 (7.3697, -198.3362) -> (7.3697, -198.8549)
  spline S87 degree 2 poles (7.3697, -198.8549) (7.2067, -198.8993) (6.8732, -198.9512) (6.7287, -198.9512) knots 0 0 0 1 2 2 2
  spline S88 degree 2 poles (8.8332, -198.9512) (8.3626, -198.9512) (7.8328, -198.414) (7.8328, -197.8323) knots 0 0 0 1 2 2 2
  line L80 (7.8328, -197.8323) -> (7.8328, -195.9316)
  line L81 (7.8328, -195.9316) -> (7.4438, -195.9316)
  line L82 (7.4438, -195.9316) -> (7.4438, -195.4537)
  line L83 (7.4438, -195.4537) -> (7.8328, -195.4537)
  line L84 (7.8328, -195.4537) -> (7.8328, -194.4681)
  line L85 (7.8328, -194.4681) -> (8.4108, -194.4681)
  line L86 (8.4108, -194.4681) -> (8.4108, -195.4537)
  line L87 (8.4108, -195.4537) -> (9.4741, -195.4537)
  line L88 (9.4741, -195.4537) -> (9.4741, -195.9316)
  line L89 (9.4741, -195.9316) -> (8.4108, -195.9316)
  line L90 (8.4108, -195.9316) -> (8.4108, -197.5655)
  spline S89 degree 2 poles (8.4108, -197.5655) (8.4108, -197.8249) (8.4293, -198.1102) (8.4923, -198.2324) knots 0 0 0 1 2 2 2
  spline S90 degree 2 poles (8.4923, -198.2324) (8.5442, -198.3399) (8.7776, -198.4473) (8.9777, -198.4473) knots 0 0 0 1 2 2 2
  spline S91 degree 2 poles (8.9777, -198.4473) (9.1185, -198.4473) (9.3815, -198.3621) (9.4408, -198.3362) knots 0 0 0 1 2 2 2
  line L91 (9.4408, -198.3362) -> (9.4741, -198.3362)
  line L92 (9.4741, -198.3362) -> (9.4741, -198.8549)
  spline S92 degree 2 poles (9.4741, -198.8549) (9.3111, -198.8993) (8.9777, -198.9512) (8.8332, -198.9512) knots 0 0 0 1 2 2 2
  spline S93 degree 2 poles (12.7197, -197.1691) (12.7197, -198.0361) (11.8861, -198.9809) (11.1896, -198.9809) knots 0 0 0 1 2 2 2
  spline S94 degree 2 poles (11.1896, -198.9809) (10.4745, -198.9809) (9.6557, -198.0064) (9.6557, -197.1691) knots 0 0 0 1 2 2 2
  spline S95 degree 2 poles (9.6557, -197.1691) (9.6557, -196.3095) (10.5004, -195.3573) (11.1896, -195.3573) knots 0 0 0 1 2 2 2
  spline S96 degree 2 poles (11.1896, -195.3573) (11.8861, -195.3573) (12.7197, -196.3058) (12.7197, -197.1691) knots 0 0 0 1 2 2 2
  spline S97 degree 2 poles (12.1232, -197.1691) (12.1232, -196.5022) (11.6379, -195.8538) (11.1896, -195.8538) knots 0 0 0 1 2 2 2
  spline S98 degree 2 poles (11.1896, -195.8538) (10.7413, -195.8538) (10.2522, -196.5022) (10.2522, -197.1691) knots 0 0 0 1 2 2 2
  spline S99 degree 2 poles (10.2522, -197.1691) (10.2522, -197.8175) (10.7413, -198.4844) (11.1896, -198.4844) knots 0 0 0 1 2 2 2
  spline S100 degree 2 poles (11.1896, -198.4844) (11.6342, -198.4844) (12.1232, -197.8286) (12.1232, -197.1691) knots 0 0 0 1 2 2 2
  line L93 (17.2028, -198.8845) -> (17.2028, -196.8986)
  spline S101 degree 2 poles (17.2028, -196.8986) (17.2028, -196.6615) (17.1658, -196.2577) (17.1065, -196.1465) knots 0 0 0 1 2 2 2
  spline S102 degree 2 poles (17.1065, -196.1465) (17.0472, -196.0242) (16.8212, -195.9057) (16.6248, -195.9057) knots 0 0 0 1 2 2 2
  spline S103 degree 2 poles (16.6248, -195.9057) (16.447, -195.9057) (16.0394, -196.1243) (15.8246, -196.3318) knots 0 0 0 1 2 2 2
  spline S104 degree 2 poles (15.8246, -196.3318) (15.8283, -196.3836) (15.8357, -196.5281) (15.8357, -196.6245) knots 0 0 0 1 2 2 2
  line L94 (15.8357, -196.6245) -> (15.8357, -198.8845)
  line L95 (15.8357, -198.8845) -> (15.2577, -198.8845)
  line L96 (15.2577, -198.8845) -> (15.2577, -196.8986)
  spline S105 degree 2 poles (15.2577, -196.8986) (15.2577, -196.6615) (15.2206, -196.2577) (15.1614, -196.1465) knots 0 0 0 1 2 2 2
  spline S106 degree 2 poles (15.1614, -196.1465) (15.1021, -196.0242) (14.8761, -195.9057) (14.6797, -195.9057) knots 0 0 0 1 2 2 2
  spline S107 degree 2 poles (14.6797, -195.9057) (14.4944, -195.9057) (14.0832, -196.1391) (13.8905, -196.3207) knots 0 0 0 1 2 2 2
  line L97 (13.8905, -196.3207) -> (13.8905, -198.8845)
  line L98 (13.8905, -198.8845) -> (13.3125, -198.8845)
  line L99 (13.3125, -198.8845) -> (13.3125, -195.4537)
  line L100 (13.3125, -195.4537) -> (13.8905, -195.4537)
  line L101 (13.8905, -195.4537) -> (13.8905, -195.8316)
  spline S108 degree 2 poles (13.8905, -195.8316) (14.1165, -195.6056) (14.5611, -195.3573) (14.8279, -195.3573) knots 0 0 0 1 2 2 2
  spline S109 degree 2 poles (14.8279, -195.3573) (15.1317, -195.3573) (15.6023, -195.6352) (15.7245, -195.9501) knots 0 0 0 1 2 2 2
  spline S110 degree 2 poles (15.7245, -195.9501) (15.9876, -195.6575) (16.484, -195.3573) (16.773, -195.3573) knots 0 0 0 1 2 2 2
  spline S111 degree 2 poles (16.773, -195.3573) (16.9953, -195.3573) (17.3584, -195.4944) (17.4918, -195.65) knots 0 0 0 1 2 2 2
  spline S112 degree 2 poles (17.4918, -195.65) (17.6289, -195.8057) (17.7808, -196.2725) (17.7808, -196.6245) knots 0 0 0 1 2 2 2
  line L102 (17.7808, -196.6245) -> (17.7808, -198.8845)
  line L103 (17.7808, -198.8845) -> (17.2028, -198.8845)
  line L104 (21.6526, -199.8034) -> (18.1254, -199.8034)
  line L105 (18.1254, -199.8034) -> (18.1254, -199.4069)
  line L106 (18.1254, -199.4069) -> (21.6526, -199.4069)
  line L107 (21.6526, -199.4069) -> (21.6526, -199.8034)
  line L108 (24.7166, -195.4537) -> (23.4236, -198.8845)
  line L109 (23.4236, -198.8845) -> (22.9049, -198.8845)
  line L110 (22.9049, -198.8845) -> (21.6229, -195.4537)
  line L111 (21.6229, -195.4537) -> (22.2491, -195.4537)
  line L112 (22.2491, -195.4537) -> (23.1864, -198.0954)
  line L113 (23.1864, -198.0954) -> (24.1164, -195.4537)
  line L114 (24.1164, -195.4537) -> (24.7166, -195.4537)
  spline S113 degree 2 poles (27.914, -196.5985) (27.914, -197.8286) (27.199, -198.9809) (26.4543, -198.9809) knots 0 0 0 1 2 2 2
  spline S114 degree 2 poles (26.4543, -198.9809) (25.6984, -198.9809) (24.9908, -197.8064) (24.9908, -196.6022) knots 0 0 0 1 2 2 2
  spline S115 degree 2 poles (24.9908, -196.6022) (24.9908, -195.3648) (25.7059, -194.2199) (26.4543, -194.2199) knots 0 0 0 1 2 2 2
  spline S116 degree 2 poles (26.4543, -194.2199) (27.2064, -194.2199) (27.914, -195.4055) (27.914, -196.5985) knots 0 0 0 1 2 2 2
  spline S117 degree 2 poles (27.1286, -197.9916) (27.2175, -197.7656) (27.2916, -197.0691) (27.2916, -196.5985) knots 0 0 0 1 2 2 2
  spline S118 degree 2 poles (27.2916, -196.5985) (27.2916, -196.128) (27.2175, -195.4352) (27.1249, -195.2017) knots 0 0 0 1 2 2 2
  spline S119 degree 2 poles (27.1249, -195.2017) (27.0323, -194.9683) (26.7099, -194.7275) (26.4543, -194.7275) knots 0 0 0 1 2 2 2
  spline S120 degree 2 poles (26.4543, -194.7275) (26.1986, -194.7275) (25.8689, -194.9683) (25.7725, -195.2091) knots 0 0 0 1 2 2 2
  spline S121 degree 2 poles (25.7725, -195.2091) (25.6799, -195.4426) (25.6132, -196.1539) (25.6132, -196.6022) knots 0 0 0 1 2 2 2
  spline S122 degree 2 poles (25.6132, -196.6022) (25.6132, -197.0839) (25.6725, -197.7286) (25.7688, -197.9805) knots 0 0 0 1 2 2 2
  spline S123 degree 2 poles (25.7688, -197.9805) (25.8578, -198.2176) (26.1875, -198.4733) (26.4543, -198.4733) knots 0 0 0 1 2 2 2
  spline S124 degree 2 poles (26.4543, -198.4733) (26.7062, -198.4733) (27.036, -198.2324) (27.1286, -197.9916) knots 0 0 0 1 2 2 2
  line L115 (29.4813, -198.8845) -> (28.7477, -198.8845)
  line L116 (28.7477, -198.8845) -> (28.7477, -198.0101)
  line L117 (28.7477, -198.0101) -> (29.4813, -198.0101)
  line L118 (29.4813, -198.0101) -> (29.4813, -198.8845)
  line L119 (33.2233, -198.8845) -> (30.4038, -198.8845)
  line L120 (30.4038, -198.8845) -> (30.4038, -198.2361)
  spline S125 degree 2 poles (30.4038, -198.2361) (30.7076, -197.9509) (31.2486, -197.421) (31.5079, -197.1358) knots 0 0 0 1 2 2 2
  spline S126 degree 2 poles (31.5079, -197.1358) (32.0303, -196.5615) (32.4119, -195.8723) (32.4119, -195.5055) knots 0 0 0 1 2 2 2
  spline S127 degree 2 poles (32.4119, -195.5055) (32.4119, -195.3129) (32.2934, -195.0239) (32.1859, -194.9313) knots 0 0 0 1 2 2 2
  spline S128 degree 2 poles (32.1859, -194.9313) (32.0785, -194.8386) (31.7969, -194.746) (31.6265, -194.746) knots 0 0 0 1 2 2 2
  spline S129 degree 2 poles (31.6265, -194.746) (31.4635, -194.746) (31.13, -194.8275) (30.9781, -194.8905) knots 0 0 0 1 2 2 2
  spline S130 degree 2 poles (30.9781, -194.8905) (30.8484, -194.9424) (30.6076, -195.0906) (30.5335, -195.1425) knots 0 0 0 1 2 2 2
  line L121 (30.5335, -195.1425) -> (30.5002, -195.1425)
  line L122 (30.5002, -195.1425) -> (30.5002, -194.4904)
  spline S131 degree 2 poles (30.5002, -194.4904) (30.6891, -194.3977) (31.3671, -194.2162) (31.6709, -194.2162) knots 0 0 0 1 2 2 2
  spline S132 degree 2 poles (31.6709, -194.2162) (32.3119, -194.2162) (33.0344, -194.8942) (33.0344, -195.4722) knots 0 0 0 1 2 2 2
  spline S133 degree 2 poles (33.0344, -195.4722) (33.0344, -195.7427) (32.9084, -196.1947) (32.7973, -196.3873) knots 0 0 0 1 2 2 2
  spline S134 degree 2 poles (32.7973, -196.3873) (32.6861, -196.5874) (32.3638, -196.9801) (32.1859, -197.1691) knots 0 0 0 1 2 2 2
  spline S135 degree 2 poles (32.1859, -197.1691) (31.8969, -197.484) (31.1893, -198.1583) (30.9781, -198.3547) knots 0 0 0 1 2 2 2
  line L123 (30.9781, -198.3547) -> (33.2233, -198.3547)
  line L124 (33.2233, -198.3547) -> (33.2233, -198.8845)
  line L125 (34.8165, -198.8845) -> (34.0829, -198.8845)
  line L126 (34.0829, -198.8845) -> (34.0829, -198.0101)
  line L127 (34.0829, -198.0101) -> (34.8165, -198.0101)
  line L128 (34.8165, -198.0101) -> (34.8165, -198.8845)
  line L129 (38.5586, -198.8845) -> (35.7391, -198.8845)
  line L130 (35.7391, -198.8845) -> (35.7391, -198.2361)
  spline S136 degree 2 poles (35.7391, -198.2361) (36.0429, -197.9509) (36.5838, -197.421) (36.8432, -197.1358) knots 0 0 0 1 2 2 2
  spline S137 degree 2 poles (36.8432, -197.1358) (37.3656, -196.5615) (37.7472, -195.8723) (37.7472, -195.5055) knots 0 0 0 1 2 2 2
  spline S138 degree 2 poles (37.7472, -195.5055) (37.7472, -195.3129) (37.6286, -195.0239) (37.5212, -194.9313) knots 0 0 0 1 2 2 2
  spline S139 degree 2 poles (37.5212, -194.9313) (37.4137, -194.8386) (37.1321, -194.746) (36.9617, -194.746) knots 0 0 0 1 2 2 2
  spline S140 degree 2 poles (36.9617, -194.746) (36.7987, -194.746) (36.4652, -194.8275) (36.3133, -194.8905) knots 0 0 0 1 2 2 2
  spline S141 degree 2 poles (36.3133, -194.8905) (36.1837, -194.9424) (35.9428, -195.0906) (35.8687, -195.1425) knots 0 0 0 1 2 2 2
  line L131 (35.8687, -195.1425) -> (35.8354, -195.1425)
  line L132 (35.8354, -195.1425) -> (35.8354, -194.4904)
  spline S142 degree 2 poles (35.8354, -194.4904) (36.0243, -194.3977) (36.7024, -194.2162) (37.0062, -194.2162) knots 0 0 0 1 2 2 2
  spline S143 degree 2 poles (37.0062, -194.2162) (37.6471, -194.2162) (38.3696, -194.8942) (38.3696, -195.4722) knots 0 0 0 1 2 2 2
  spline S144 degree 2 poles (38.3696, -195.4722) (38.3696, -195.7427) (38.2437, -196.1947) (38.1325, -196.3873) knots 0 0 0 1 2 2 2
  spline S145 degree 2 poles (38.1325, -196.3873) (38.0214, -196.5874) (37.699, -196.9801) (37.5212, -197.1691) knots 0 0 0 1 2 2 2
  spline S146 degree 2 poles (37.5212, -197.1691) (37.2322, -197.484) (36.5245, -198.1583) (36.3133, -198.3547) knots 0 0 0 1 2 2 2
  line L133 (36.3133, -198.3547) -> (38.5586, -198.3547)
  line L134 (38.5586, -198.3547) -> (38.5586, -198.8845)
  spline S147 degree 2 poles (7.3067, -204.9302) (7.3067, -205.2822) (7.0733, -205.8787) (6.8769, -206.0788) knots 0 0 0 1 2 2 2
  spline S148 degree 2 poles (6.8769, -206.0788) (6.6731, -206.2899) (6.1619, -206.5085) (5.8543, -206.5085) knots 0 0 0 1 2 2 2
  spline S149 degree 2 poles (5.8543, -206.5085) (5.5468, -206.5085) (5.0392, -206.3011) (4.8466, -206.0936) knots 0 0 0 1 2 2 2
  spline S150 degree 2 poles (4.8466, -206.0936) (4.6094, -205.8453) (4.3427, -205.0117) (4.3427, -204.4041) knots 0 0 0 1 2 2 2
  spline S151 degree 2 poles (4.3427, -204.4041) (4.3427, -203.8076) (4.5872, -202.848) (4.8429, -202.4923) knots 0 0 0 1 2 2 2
  spline S152 degree 2 poles (4.8429, -202.4923) (5.0911, -202.144) (5.8766, -201.755) (6.3916, -201.755) knots 0 0 0 1 2 2 2
  spline S153 degree 2 poles (6.3916, -201.755) (6.5435, -201.755) (6.8102, -201.7846) (6.9103, -201.818) knots 0 0 0 1 2 2 2
  line L135 (6.9103, -201.818) -> (6.9103, -202.4071)
  line L136 (6.9103, -202.4071) -> (6.8843, -202.4071)
  spline S154 degree 2 poles (6.8843, -202.4071) (6.7991, -202.3626) (6.4879, -202.2848) (6.3101, -202.2848) knots 0 0 0 1 2 2 2
  spline S155 degree 2 poles (6.3101, -202.2848) (5.7395, -202.2848) (5.0392, -203.0555) (4.9725, -203.8113) knots 0 0 0 1 2 2 2
  spline S156 degree 2 poles (4.9725, -203.8113) (5.1911, -203.6594) (5.6506, -203.4926) (5.9247, -203.4926) knots 0 0 0 1 2 2 2
  spline S157 degree 2 poles (5.9247, -203.4926) (6.1915, -203.4926) (6.5916, -203.6001) (6.8102, -203.7631) knots 0 0 0 1 2 2 2
  spline S158 degree 2 poles (6.8102, -203.7631) (7.0622, -203.9521) (7.3067, -204.5375) (7.3067, -204.9302) knots 0 0 0 1 2 2 2
  spline S159 degree 2 poles (6.6843, -204.9561) (6.6843, -204.6745) (6.5361, -204.2929) (6.373, -204.1596) knots 0 0 0 1 2 2 2
  spline S160 degree 2 poles (6.373, -204.1596) (6.2508, -204.0632) (5.947, -204.0002) (5.7876, -204.0002) knots 0 0 0 1 2 2 2
  spline S161 degree 2 poles (5.7876, -204.0002) (5.5728, -204.0002) (5.1689, -204.1299) (4.9725, -204.2522) knots 0 0 0 1 2 2 2
  spline S162 degree 2 poles (4.9725, -204.2522) (4.9688, -204.3189) (4.9614, -204.4448) (4.9614, -204.5412) knots 0 0 0 1 2 2 2
  spline S163 degree 2 poles (4.9614, -204.5412) (4.9614, -205.0154) (5.1467, -205.5971) (5.2875, -205.749) knots 0 0 0 1 2 2 2
  spline S164 degree 2 poles (5.2875, -205.749) (5.4171, -205.8935) (5.6987, -206.0084) (5.858, -206.0084) knots 0 0 0 1 2 2 2
  spline S165 degree 2 poles (5.858, -206.0084) (6.2285, -206.0084) (6.6843, -205.4822) (6.6843, -204.9561) knots 0 0 0 1 2 2 2
  line L137 (9.7483, -201.6364) -> (7.9588, -207.4052)
  line L138 (7.9588, -207.4052) -> (7.4401, -207.4052)
  line L139 (7.4401, -207.4052) -> (9.2222, -201.6364)
  line L140 (9.2222, -201.6364) -> (9.7483, -201.6364)
  line L141 (13.0717, -206.4122) -> (10.2522, -206.4122)
  line L142 (10.2522, -206.4122) -> (10.2522, -205.7638)
  spline S166 degree 2 poles (10.2522, -205.7638) (10.556, -205.4785) (11.0969, -204.9487) (11.3563, -204.6634) knots 0 0 0 1 2 2 2
  spline S167 degree 2 poles (11.3563, -204.6634) (11.8787, -204.0892) (12.2603, -203.4) (12.2603, -203.0332) knots 0 0 0 1 2 2 2
  spline S168 degree 2 poles (12.2603, -203.0332) (12.2603, -202.8406) (12.1418, -202.5516) (12.0343, -202.4589) knots 0 0 0 1 2 2 2
  spline S169 degree 2 poles (12.0343, -202.4589) (11.9269, -202.3663) (11.6453, -202.2737) (11.4749, -202.2737) knots 0 0 0 1 2 2 2
  spline S170 degree 2 poles (11.4749, -202.2737) (11.3118, -202.2737) (10.9784, -202.3552) (10.8265, -202.4182) knots 0 0 0 1 2 2 2
  spline S171 degree 2 poles (10.8265, -202.4182) (10.6968, -202.4701) (10.456, -202.6183) (10.3819, -202.6701) knots 0 0 0 1 2 2 2
  line L143 (10.3819, -202.6701) -> (10.3485, -202.6701)